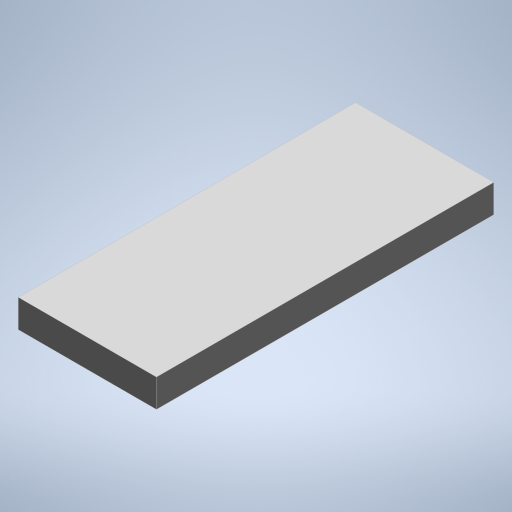
# Autodesk Inventor part: Table
Saved by Autodesk Inventor 2023 (Build 270158000, 158)
## iProperties
Created: 2021-10-07
Part Number: Table
Material: Generic
Document SubType Name: Modeling
Designer: gnzak
Density: 1 g/cm^3
Appearance: Dark Gray
Author: gnzak
Autodesk Inventor part; units mm, degrees
ref_plane "YZ Plane" through (0, 0, 0) normal (1, 0, 0) x (0, 1, 0)
sketch "Sketch1" plane through (0, 0, 0) normal (0, 1, 0) x (-1, 0, 0)
  line L0 (749.3, 1828.8) -> (-749.3, 1828.8)
  line L1 (-749.3, 1828.8) -> (-749.3, -1828.8)
  line L2 (-749.3, -1828.8) -> (749.3, -1828.8)
  line L3 (749.3, -1828.8) -> (749.3, 1828.8)
  point P0 (0, 0)
  dimension "d0" = 749.3
  dimension "d1" = 1828.8
  dimension "d2" = 3657.6
  dimension "d3" = 1498.6
  constraints: 8 end point, 2 parallel, 1 horizontal, 1 perpendicular
  measures "d0" distance from line of L3 point (0, 0)
  measures "d1" distance from line of point (0, 0) L0
  measures "d2" distance of L0.end L1.end
  measures "d3" distance of L0.start L0.end
extrude "Extrusion1" add sketch "Sketch1" along normal blind 304.8
sketch "Sketch2" plane through (0, 304.8, 0) normal (0, 1, 0) x (1, 0, 0)
  line L0 (-749.3, -1828.8) -> (749.3, -1828.8) projected
  line L1 (-749.3, 1828.8) -> (-749.3, -1828.8) projected
  line L2 (-749.3, -1816.1) -> (749.3, -1816.1)
  line L3 (0, -1816.1) -> (0, -1188.3136)
  point P0 (0, 0)
  dimension "d7" = 12.7
  dimension "d8" = 1498.6
  dimension "d9" = 627.7864
  constraints: 4 end point, 1 coincident, 1 horizontal, 1 midpoint, 1 point on line, 1 vertical
  measures "d7" distance between parallel lines of L0 L2
  measures "d8" distance of L2.start L2.end
  measures "d9" distance of L3.start L3.end
ref_plane "Work Plane1" through (0, 304.8, 1188.3136) normal (0, 0, 1) x (1, 0, 0)
ref_plane "Work Plane2" through (0, 0, -1828.8) normal (-1, 0, 0) x (0, 0, 1)
equation "\"d0\" = 0.5 * d3"
equation "\"d1\" = 0.5 * d2"
body "Solid1"
